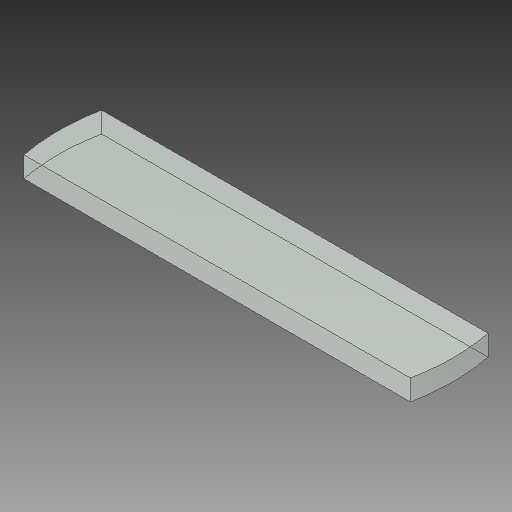
# Autodesk Inventor part: Rotor
Saved by Autodesk Inventor 2018 (Build 220112000, 112)
## iProperties
Created: 2017-12-31
Part Number: Rotor
Material: Generic
Document SubType Name: Modeling
Designer: suchanek
Density: 1 g/cm^3
Appearance: Default
Mass: 4.5423 g
Surface Area: 29.8961 cm^2
Volume: 4.5423 cm^3
Author: suchanek
Autodesk Inventor part; units mm, degrees
ref_plane "YZ Plane" through (0, 0, 0) normal (1, 0, 0) x (0, 1, 0)
ref_plane "XZ Plane" through (0, 0, 0) normal (0, 1, 0) x (-1, 0, 0)
ref_plane "XY Plane" through (0, 0, 0) normal (0, 0, 1) x (1, 0, 0)
sketch "Sketch1" plane through (0, 0, 0) normal (0, 1, 0) x (-1, 0, 0)
  circle A0 centre (0, 0) radius 38.1
  dimension "d0" = 76.2
  constraints: 1 centre point, 1 coincident
  measures "d0" diameter of A0
extrude "Extrusion1" add sketch "Sketch1" along normal blind 4
sketch "Sketch2" plane through (0, 0, 0) normal (0, -1, 0) x (1, 0, 0)
  line L0 (-50, 7.5) -> (50, 7.5)
  line L1 (50, 7.5) -> (50, -7.5)
  line L2 (50, -7.5) -> (-50, -7.5)
  line L3 (-50, -7.5) -> (-50, 7.5)
  point P0 (0, 0)
  dimension "d3" = 15
  dimension "d4" = 7.5
  dimension "d5" = 100
  dimension "d6" = 50
  constraints: 8 end point, 2 parallel, 1 horizontal, 1 perpendicular
  measures "d3" distance between parallel lines of L0 L2
  measures "d4" distance from line of L0 point (0, 0)
  measures "d5" distance between parallel lines of L1 L3
  measures "d6" distance from line of point (0, 0) L3
extrude "Extrusion2" cut sketch "Sketch2" against normal blind 10 keep common part
body "Solid1"
